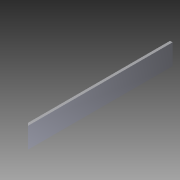
# Autodesk Inventor part: left frame peace 2
Saved by Autodesk Inventor 2012 (Build 160160000, 160)
## iProperties
Created: 2013-01-04
Part Number: left frame peace 2
Material: Default
Document SubType Name: Modeling
Designer: Bryce
Density: 1 g/cm^3
Author: Bryce
Autodesk Inventor part; units mm, degrees
ref_plane "YZ Plane" through (0, 0, 0) normal (1, 0, 0) x (0, 1, 0)
ref_plane "XZ Plane" through (0, 0, 0) normal (0, 1, 0) x (-1, 0, 0)
ref_plane "XY Plane" through (0, 0, 0) normal (0, 0, 1) x (1, 0, 0)
sketch "Sketch1" plane through (0, 0, 0) normal (0, 0, 1) x (1, 0, 0)
  line L0 (0, 0) -> (0, 25.4)
  line L1 (0, 0) -> (25.4, 0)
  line L2 (25.4, 0) -> (25.4, 3.175)
  line L3 (25.4, 3.175) -> (3.175, 3.175)
  line L4 (3.175, 3.175) -> (3.175, 25.4)
  line L5 (3.175, 25.4) -> (0, 25.4)
  dimension "d0" = 25.4
  dimension "d1" = 25.4
  dimension "d2" = 3.175
  dimension "d3" = 3.175
  constraints: 12 end point, 2 parallel, 2 perpendicular, 2 vertical
  measures "d0" distance of L0.start L0.end
  measures "d1" distance of L0.start L1.end
  measures "d2" distance between parallel lines of L4 L0
  measures "d3" distance between parallel lines of L1 L3
extrude "Extrusion1" add sketch "Sketch1" along normal blind 177.8
sketch "Sketch2" plane through (0, 0, 0) normal (0, -1, 0) x (1, 0, 0)
  line L0 (25.4, 177.8) -> (0, 177.8) projected
  line L1 (25.4, 0) -> (25.4, 177.8) projected
  line L2 (0, 177.8) -> (25.4, 152.4)
  circle A0 centre (12.7, 136.525) radius 3.175
  circle A1 centre (12.7, 60.325) radius 3.175
  dimension "d6" = 45
  dimension "d7" = 41.275
  dimension "d8" = 76.2
  dimension "d9" = 6.35
  dimension "d10" = 12.7
  constraints: 2 centre point, 2 end point, 1 equal radius, 1 point on line, 1 vertical alignment
  measures "d6" angle of L0 L2
  measures "d7" vertical distance of A0.centre L0.end
  measures "d8" distance of A1.centre A0.centre
  measures "d9" diameter of A0
  measures "d10" distance from line of L1 A0.centre
extrude "Extrusion2" cut sketch "Sketch2" against normal through all
mirror "Mirror1" about plane through (25.4, 3.175, 0) normal (1, 0, 0) remove original yes
body "Solid1"
